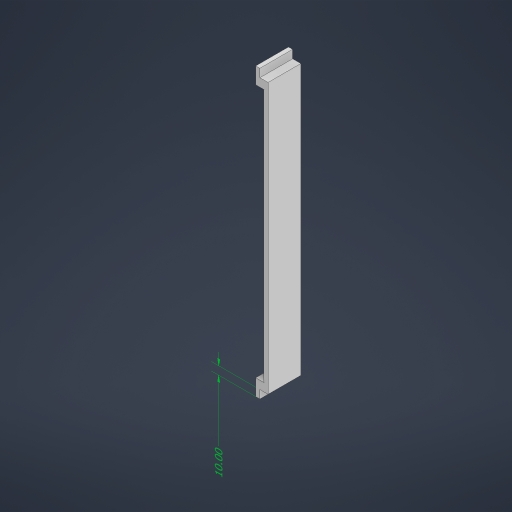
# Autodesk Inventor part: link
Saved by Autodesk Inventor 2024 (Build 280153000, 153)
## iProperties
Created: 2023-06-19
Part Number: link
Material: 일반
Document SubType Name: Modeling
Designer: 6gioc
Density: 1 g/cm^3
Appearance: 기본값
Author: 6gioc
Autodesk Inventor part; units mm, degrees
ref_plane "YZ Plane" through (0, 0, 0) normal (1, 0, 0) x (0, 1, 0)
ref_plane "XZ Plane" through (0, 0, 0) normal (0, 1, 0) x (-1, 0, 0)
ref_plane "XY Plane" through (0, 0, 0) normal (0, 0, 1) x (1, 0, 0)
sketch "스케치1" plane through (0, 0, 0) normal (1, 0, 0) x (0, 1, 0)
  line L0 (0, 0) -> (20, 0)
  line L1 (20, 0) -> (20, -40)
  line L2 (20, -40) -> (0, -40)
  line L3 (0, -40) -> (0, 0)
  dimension "d0" = 20
  dimension "d1" = 40
  constraints: 8 end point, 2 parallel, 1 horizontal, 1 perpendicular
  measures "d0" distance of L1.end L2.end
  measures "d1" distance of L0.end L1.end
extrude "돌출1" add sketch "스케치1" along normal blind 5
sketch "스케치2" plane through (5, 0, 0) normal (1, 0, 0) x (0, 0, -1)
  line L0 (40, 20) -> (0, 20) projected
  line L1 (0, 20) -> (40, 20)
  line L2 (40, 20) -> (40, 10)
  line L3 (40, 10) -> (0, 10)
  line L4 (0, 10) -> (0, 20)
  point P0 (0, 0)
  dimension "d4" = 40
  dimension "d5" = 10
  constraints: 8 end point, 2 parallel, 1 horizontal, 1 perpendicular
  measures "d4" distance of L2.end L3.end
  measures "d5" distance of L1.end L2.end
extrude "돌출2" add sketch "스케치2" along normal blind 10
sketch "스케치3" plane through (15, 0, 0) normal (1, 0, 0) x (0, 0, -1)
  line L0 (0, 20) -> (40, 20)
  line L1 (40, 20) -> (40, 330)
  line L2 (40, 330) -> (0, 330)
  line L3 (0, 330) -> (0, 20)
  line L4 (40, 20) -> (0, 20) projected
  point P0 (0, 0)
  dimension "d8" = 40
  dimension "d9" = 310
  constraints: 8 end point, 3 equal length, 1 collinear, 1 horizontal, 1 perpendicular
  measures "d8" distance of L2.end L1.end
  measures "d9" distance of L1.end L0.end
extrude "돌출3" add sketch "스케치3" against normal blind 5
sketch "스케치4" plane through (15, 330, 0) normal (0, 1, 0) x (1, 0, 0)
  line L0 (0, 0) -> (0, 40) projected
  line L1 (-15, 40) -> (-15, 0) projected
  line L2 (0, 0) -> (-15, 0)
  line L3 (-15, 0) -> (-15, 40)
  line L4 (-15, 40) -> (0, 40)
  line L5 (0, 40) -> (0, 0)
  dimension "d15" = 15
  dimension "d16" = 40
  constraints: 8 end point, 2 parallel, 1 horizontal, 1 perpendicular
  measures "d15" distance of L1.start L4.end
  measures "d16" distance of L2.end L1.start
extrude "돌출4" add sketch "스케치4" along normal blind 10
sketch "스케치5" plane through (15, 340, 0) normal (0, 1, 0) x (1, 0, 0)
  line L0 (-15, 40) -> (-10, 40) projected
  line L1 (-15, 40) -> (-10, 40)
  line L2 (-10, 40) -> (-10, 0)
  line L3 (-10, 0) -> (-15, 0)
  line L4 (-15, 0) -> (-15, 40)
  dimension "d19" = 5
  dimension "d20" = 40
  constraints: 8 end point, 2 parallel, 1 horizontal, 1 perpendicular
  measures "d19" distance of L2.end L3.end
  measures "d20" distance of L1.end L2.end
extrude "돌출5" add sketch "스케치5" along normal blind 10
